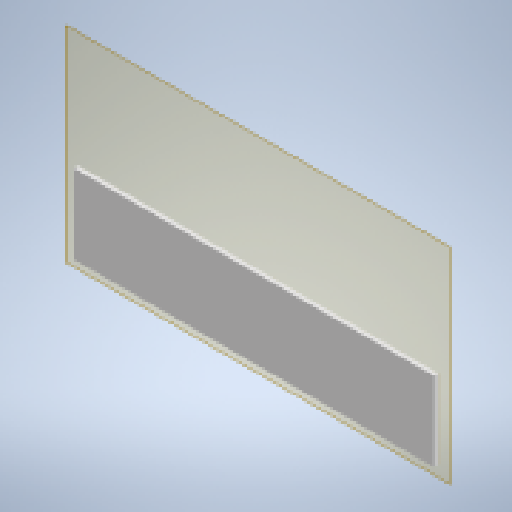
# Autodesk Inventor part: slider
Saved by Autodesk Inventor 2025 (Build 290162010, 162A)
## iProperties
Created: 2024-06-17
Part Number: slider
Material: 일반
Document SubType Name: Modeling
Designer: user
Density: 1 g/cm^3
Appearance: 기본값
Author: user
Autodesk Inventor part; units mm, degrees
ref_plane "YZ Plane" through (0, 0, 0) normal (1, 0, 0) x (0, 1, 0)
ref_plane "XZ Plane" through (0, 0, 0) normal (0, 1, 0) x (-1, 0, 0)
ref_plane "XY Plane" through (0, 0, 0) normal (0, 0, 1) x (1, 0, 0)
ref_plane "작업 평면1" through (0, -81.1446, -7162) normal (0, 0, 1) x (1, 0, 0)
sketch "스케치1" plane through (0, -81.1446, -7162) normal (0, 0, 1) x (1, 0, 0)
  line L0 (-329.749, -159.2005) -> (330.251, -159.2005)
  line L1 (330.251, -159.2005) -> (330.251, -14.2005)
  line L2 (330.251, -14.2005) -> (-329.749, -14.2005)
  line L3 (-329.749, -14.2005) -> (-329.749, -159.2005)
  point P0 (0, 81.1446)
  dimension "d0" = 660
  dimension "d1" = 145
  constraints: 8 end point, 2 parallel, 1 horizontal, 1 perpendicular
  measures "d0" distance of L2.end L1.end
  measures "d1" distance of L1.end L0.end
extrude "돌출1" add sketch "스케치1" along normal blind 8
sketch "스케치3" plane through (-329.749, -240.3451, -7162) normal (-1, 0, 0) x (0, 0, 1)
  line L0 (0, 0) -> (0, 145) projected
  line L1 (0, 145) -> (8, 145) projected
  line L2 (0, 0) -> (4, 0)
  line L3 (4, 0) -> (4, 145)
  line L4 (4, 145) -> (0, 145)
  line L5 (0, 145) -> (0, 0)
  point P0 (7162, 240.3451)
  constraints: 8 end point, 2 parallel, 1 horizontal, 1 midpoint, 1 perpendicular
extrude "돌출2" add sketch "스케치3" along normal blind 5
sketch "스케치4" plane through (330.251, -240.3451, -7162) normal (1, 0, 0) x (0, 0, -1)
  line L0 (0, 0) -> (0, 145) projected
  line L1 (0, 0) -> (-8, 0) projected
  line L2 (0, 145) -> (-4, 145)
  line L3 (-4, 145) -> (-4, 0)
  line L4 (-4, 0) -> (0, 0)
  line L5 (0, 0) -> (0, 145)
  point P0 (-7162, 240.3451)
  constraints: 8 end point, 2 parallel, 1 horizontal, 1 midpoint, 1 perpendicular
extrude "돌출3" add sketch "스케치4" along normal blind 5
